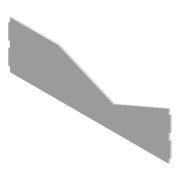
# Autodesk Inventor part: Fondo
Saved by Autodesk Inventor 2022 (Build 260153000, 153)
## iProperties
Created: 2022-06-06
Part Number: Fondo
Material: Generic
Document SubType Name: Modeling
Designer: ADMIN
Density: 1 g/cm^3
Appearance: Default
Author: ADMIN
Autodesk Inventor part; units mm, degrees
ref_plane "YZ Plane" through (0, 0, 0) normal (1, 0, 0) x (0, 1, 0)
ref_plane "XZ Plane" through (0, 0, 0) normal (0, 1, 0) x (-1, 0, 0)
ref_plane "XY Plane" through (0, 0, 0) normal (0, 0, 1) x (1, 0, 0)
sketch "Sketch1" plane through (0, 0, 0) normal (0, 0, 1) x (1, 0, 0)
  line L0 (250, -75) -> (-250, -75) projected
  line L1 (250, 75) -> (250, -75) projected
  line L2 (75, 0) -> (250, 75) projected
  line L3 (-100, 75) -> (75, 0) projected
  line L4 (-250, 75) -> (-100, 75) projected
  line L5 (-250, -75) -> (-250, 75) projected
  line L6 (-255, -10) -> (-255, -60) projected
  line L7 (-255, -60) -> (-250, -60) projected
  line L8 (-250, -10) -> (-250, -60) projected
  line L9 (-255, -10) -> (-250, -10) projected
  line L10 (-255, 60) -> (-255, 10) projected
  line L11 (-255, 10) -> (-250, 10) projected
  line L12 (-250, 60) -> (-250, 10) projected
  line L13 (-255, 60) -> (-250, 60) projected
  line L14 (250, 60) -> (250, 10) projected
  line L15 (250, 10) -> (255, 10) projected
  line L16 (255, 60) -> (255, 10) projected
  line L17 (250, 60) -> (255, 60) projected
  line L18 (250, -10) -> (250, -60) projected
  line L19 (250, -60) -> (255, -60) projected
  line L20 (255, -10) -> (255, -60) projected
  line L21 (250, -10) -> (255, -10) projected
  point P0 (0, 0)
extrude "Extrusion1" add sketch "Sketch1" along normal blind 5
sketch "Sketch2" plane through (0, 0, 5) normal (0, 0, 1) x (1, 0, 0)
  point P0 (0, 0)
sketch "Sketch3" plane through (0, 0, 5) normal (0, 0, 1) x (1, 0, 0)
  line L0 (27.0732, 15.1002) -> (29.0427, 19.696) projected
  line L1 (29.0427, 19.696) -> (75, 0) projected
  line L2 (75, 0) -> (120.9573, 19.696) projected
  line L3 (120.9573, 19.696) -> (122.9268, 15.1002) projected
  line L4 (122.9268, 15.1002) -> (150.5012, 26.9178) projected
  line L5 (150.5012, 26.9178) -> (148.5316, 31.5135) projected
  line L6 (148.5316, 31.5135) -> (176.106, 43.3311) projected
  line L7 (176.106, 43.3311) -> (178.0755, 38.7354) projected
  line L8 (178.0755, 38.7354) -> (205.6499, 50.553) projected
  line L9 (205.6499, 50.553) -> (203.6803, 55.1487) projected
  line L10 (203.6803, 55.1487) -> (250, 75) projected
  line L11 (250, 75) -> (250, 60) projected
  line L12 (250, 60) -> (255, 60) projected
  line L13 (255, 60) -> (255, 10) projected
  line L14 (255, 10) -> (250, 10) projected
  line L15 (250, 10) -> (250, -10) projected
  line L16 (250, -10) -> (255, -10) projected
  line L17 (255, -10) -> (255, -60) projected
  line L18 (255, -60) -> (250, -60) projected
  line L19 (250, -60) -> (250, -75) projected
  line L20 (250, -75) -> (-250, -75) projected
  line L21 (-250, -75) -> (-250, -60) projected
  line L22 (-250, -60) -> (-255, -60) projected
  line L23 (-255, -60) -> (-255, -10) projected
  line L24 (-255, -10) -> (-250, -10) projected
  line L25 (-250, -10) -> (-250, 10) projected
  line L26 (-250, 10) -> (-255, 10) projected
  line L27 (-255, 10) -> (-255, 60) projected
  line L28 (-255, 60) -> (-250, 60) projected
  line L29 (-250, 60) -> (-250, 75) projected
  line L30 (-250, 75) -> (-220, 75) projected
  line L31 (-220, 75) -> (-220, 70) projected
  line L32 (-220, 70) -> (-190, 70) projected
  line L33 (-190, 70) -> (-190, 75) projected
  line L34 (-190, 75) -> (-160, 75) projected
  line L35 (-160, 75) -> (-160, 70) projected
  line L36 (-160, 70) -> (-130, 70) projected
  line L37 (-130, 70) -> (-130, 75) projected
  line L38 (-130, 75) -> (-100, 75) projected
  line L39 (-100, 75) -> (-53.6803, 55.1487) projected
  line L40 (-53.6803, 55.1487) -> (-55.6499, 50.553) projected
  line L41 (-55.6499, 50.553) -> (-28.0755, 38.7354) projected
  line L42 (-28.0755, 38.7354) -> (-26.106, 43.3311) projected
  line L43 (-26.106, 43.3311) -> (1.4684, 31.5135) projected
  line L44 (1.4684, 31.5135) -> (-0.5012, 26.9178) projected
  line L45 (-0.5012, 26.9178) -> (27.0732, 15.1002) projected
  line L46 (-255, 10) -> (-250, 10) projected
  line L47 (-250, 10) -> (-250, -10) projected
  line L48 (-250, -10) -> (-255, -10) projected
  line L49 (-255, -10) -> (-255, -60) projected
  line L50 (-255, -60) -> (-250, -60) projected
  line L51 (-250, -60) -> (-250, -75) projected
  line L52 (-250, -75) -> (250, -75) projected
  line L53 (250, -75) -> (250, -60) projected
  line L54 (250, -60) -> (255, -60) projected
  line L55 (255, -60) -> (255, -10) projected
  line L56 (255, -10) -> (250, -10) projected
  line L57 (250, -10) -> (250, 10) projected
  line L58 (250, 10) -> (255, 10) projected
  line L59 (255, 10) -> (255, 60) projected
  line L60 (255, 60) -> (250, 60) projected
  line L61 (250, 60) -> (250, 75) projected
  line L62 (250, 75) -> (75, 0) projected
  line L63 (75, 0) -> (-100, 75) projected
  line L64 (-100, 75) -> (-250, 75) projected
  line L65 (-250, 75) -> (-250, 60) projected
  line L66 (-250, 60) -> (-255, 60) projected
  line L67 (-255, 60) -> (-255, 10) projected
  line L68 (-220, 10) -> (-220, 5) projected
  line L69 (-220, 5) -> (-190, 5) projected
  line L70 (-190, 5) -> (-190, 10) projected
  line L71 (-190, 10) -> (-220, 10) projected
  line L72 (-160, 10) -> (-160, 5) projected
  line L73 (-160, 5) -> (-130, 5) projected
  line L74 (-130, 5) -> (-130, 10) projected
  line L75 (-130, 10) -> (-160, 10) projected
  point P0 (0, 0)
extrude "Extrusion2" cut sketch "Sketch3" against normal blind 5 contours L45 L44 L63 L0 | L62 L5 L4 L3 | L42 L41 L40 L63 | L62 L9 L8 L7 | L37 L36 L35 L64 | L33 L32 L31 L64
body "Solid1"
